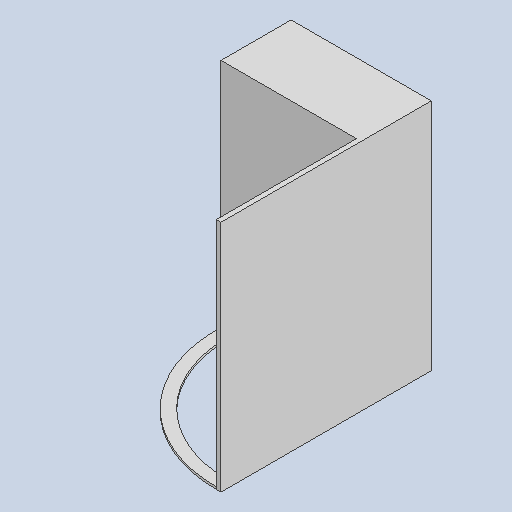
# Autodesk Inventor part: Electrical box 2
Saved by Autodesk Inventor 2025.4 (Build 294407000, 407)
## iProperties
Created: 2026-01-26
Part Number: Electrical box 2
Material: Generic
Document SubType Name: Modeling
Designer: admin
Density: 1 g/cm^3
Appearance: Default
Author: admin
Autodesk Inventor part; units mm, degrees
ref_plane "YZ Plane" through (0, 0, 0) normal (1, 0, 0) x (0, 1, 0)
ref_plane "XZ Plane" through (0, 0, 0) normal (0, 1, 0) x (-1, 0, 0)
ref_plane "XY Plane" through (0, 0, 0) normal (0, 0, 1) x (1, 0, 0)
sketch "Sketch1" plane through (0, 0, 0) normal (0, 1, 0) x (-1, 0, 0)
  line L0 (0, 0) -> (-600, 0)
  line L1 (-600, 0) -> (-600, 300)
  line L2 (-600, 300) -> (0, 300)
  line L3 (0, 300) -> (0, 0)
  line L4 (0, 300) -> (-20, 300)
  line L5 (-600, 300) -> (-580, 300)
  line L6 (-580, 300) -> (-580, 900)
  line L7 (-580, 900) -> (-600, 900)
  line L8 (-600, 900) -> (-600, 300)
  dimension "d0" = 600
  dimension "d1" = 300
  dimension "d9" = 600
  dimension "d10" = 20
  constraints: 18 end point, 4 parallel, 3 horizontal, 2 perpendicular
  measures "d0" distance of L0.start L0.end
  measures "d1" distance of L2.end L0.start
  measures "d9" distance of L7.end L1.end
  measures "d10" distance of L6.end L7.end
extrude "Extrusion1" add sketch "Sketch1" along normal blind 1000
sketch "Sketch3" plane through (0, 0, 0) normal (0, 1, 0) x (-1, 0, 0)
  line L0 (0, 300) -> (-580, 300) projected
  line L1 (-580, 300) -> (-580, 900) projected
  line L2 (-580, 900) -> (-600, 900) projected
  line L3 (-600, 900) -> (-600, 0) projected
  line L4 (-600, 0) -> (0, 0) projected
  line L5 (0, 0) -> (0, 300) projected
  arc A0 (0, 300) -> (-580, 900) centre (-580, 319.6667) ccw
  arc A1 (-50.0314, 300) -> (-580, 850) centre (-580, 319.6667) ccw
  dimension "d11" = 50
  constraints: 4 point on circle, 3 point on line, 2 centre point
  measures "d11" radial gap between concentric circles of A0 A1
extrude "Extrusion3" add sketch "Sketch3" along normal blind 10 contours L0 A1 L1 A0
equation "\"d9\" = d0"
body "Solid1"
